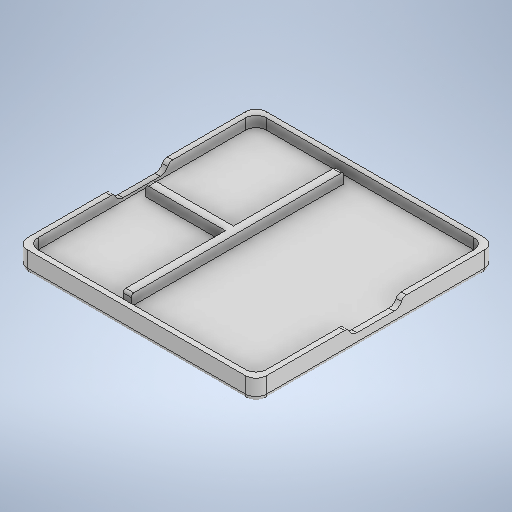
# Autodesk Inventor part: box-2
Saved by Autodesk Inventor 2025 (Build 290162000, 162)
## iProperties
Created: 2026-01-27
Part Number: box-2
Material: 一般
Document SubType Name: Modeling
Designer: mahhy
Density: 1 g/cm^3
Appearance: 既定
Author: mahhy
## iProperties of the stored document box-2_3D プリント.ipt
Created: 2026-01-27
Part Number: box-2_3D プリント
Material: 一般
Document SubType Name: Modeling
Designer: mahhy
Density: 1 g/cm^3
Appearance: 既定
Author: mahhy
Autodesk Inventor part; units mm, degrees
ref_plane "YZ Plane" through (0, 0, 0) normal (1, 0, 0) x (0, 1, 0)
ref_plane "XZ Plane" through (0, 0, 0) normal (0, 1, 0) x (-1, 0, 0)
ref_plane "XY Plane" through (0, 0, 0) normal (0, 0, 1) x (1, 0, 0)
sketch "底面スケッチ" plane through (0, 0, 0) normal (0, 1, 0) x (-1, 0, 0)
  line L0 (2, 0) -> (43, 0)
  line L1 (45, -2) -> (45, -43)
  line L2 (43, -45) -> (2, -45)
  line L3 (0, -43) -> (0, -2)
  arc A0 (45, -2) -> (43, 0) centre (43, -2) ccw
  arc A1 (43, -45) -> (45, -43) centre (43, -43) ccw
  arc A2 (0, -43) -> (2, -45) centre (2, -43) ccw
  arc A3 (2, 0) -> (0, -2) centre (2, -2) ccw
  point P0 (0, 0)
  point P1 (45, -45)
  point P2 (45, 0)
  point P3 (0, -45)
  dimension "d0" = 45
  dimension "d1" = 45
  dimension "d4" = 2
  constraints: 8 end point, 8 point on circle, 8 point on line, 8 tangent, 4 centre point, 3 equal radius, 2 parallel, 1 horizontal, 1 perpendicular
  measures "d0" distance of point (45, -45) point (0, -45)
  measures "d1" distance between parallel lines of L2 L0
  measures "d4" radius of A0
extrude "押し出し1" add sketch "底面スケッチ" along normal blind 4
sketch "スケッチ2" plane through (0, 4, 0) normal (0, 1, 0) x (1, 0, 0)
  line L0 (-42, 1) -> (-3, 1)
  line L1 (-1, 3) -> (-1, 42)
  line L2 (-3, 44) -> (-42, 44)
  line L3 (-44, 42) -> (-44, 3)
  line L4 (-2, 45) -> (-43, 45) projected
  line L5 (-43, 0) -> (-2, 0) projected
  line L6 (-45, 43) -> (-45, 2) projected
  line L7 (0, 2) -> (0, 43) projected
  arc A0 (-44, 3) -> (-42, 1) centre (-42, 3) ccw
  arc A1 (-3, 1) -> (-1, 3) centre (-3, 3) ccw
  arc A2 (-42, 44) -> (-44, 42) centre (-42, 42) ccw
  arc A3 (-1, 42) -> (-3, 44) centre (-3, 42) ccw
  point P0 (0, 0)
  dimension "d5" = 1
  dimension "d6" = 1
  dimension "d7" = 1
  dimension "d8" = 1
  dimension "d9" = 2
  constraints: 8 end point, 8 point on circle, 8 tangent, 4 centre point, 3 equal radius, 2 parallel, 1 horizontal, 1 perpendicular
  measures "d5" distance between parallel lines of L4 L2
  measures "d6" distance between parallel lines of L5 L0
  measures "d7" distance between parallel lines of L6 L3
  measures "d8" distance between parallel lines of L7 L1
  measures "d9" radius of A0
extrude "押し出し2" cut sketch "スケッチ2" against normal blind 2
sketch "スケッチ3" plane through (0, 2, 0) normal (0, 1, 0) x (1, 0, 0)
  line L0 (-3, 1) -> (-42, 1) projected
  line L1 (-42, 44) -> (-3, 44) projected
  line L2 (-44, 3) -> (-44, 42) projected
  line L3 (-27.5, 2.5) -> (-26, 2.5)
  line L4 (-26, 2.5) -> (-26, 42.5)
  line L5 (-26, 42.5) -> (-27.5, 42.5)
  line L6 (-27.5, 42.5) -> (-27.5, 2.5)
  line L7 (-1, 42) -> (-1, 3) projected
  line L8 (-27.5, 21.75) -> (-42.5, 21.75)
  line L9 (-42.5, 21.75) -> (-42.5, 23.25)
  line L10 (-42.5, 23.25) -> (-27.5, 23.25)
  line L11 (-27.5, 23.25) -> (-27.5, 21.75)
  point P0 (0, 0)
  point P1 (-26, 22.5)
  point P2 (-1, 22.5)
  point P3 (-42.5, 22.5)
  point P4 (-1, 22.5)
  dimension "d19" = 1.5
  dimension "d20" = 40
  dimension "d21" = 16.5
  dimension "d22" = 1.5
  dimension "d23" = 15
  constraints: 16 end point, 4 midpoint, 4 parallel, 2 horizontal, 2 horizontal alignment, 2 perpendicular, 1 point on line
  measures "d19" distance of L5.end L4.end
  measures "d20" distance of L3.end L4.end
  measures "d21" distance between parallel lines of L2 L6
  measures "d22" distance of L8.end L9.end
  measures "d23" distance of L9.end L10.end
extrude "押し出し3" add sketch "スケッチ3" along normal blind 2
fillet "フィレット1" radius 0.5 3 edges at (-26.75, 4, -42.5) (-26.75, 4, -2.5) (-42.5, 4, -22.5)
fillet "フィレット2" radius 1 8 edges at (-44.4142, 0, -44.4142) (-45, 0, -22.5) (-44.4142, 0, -0.5858) (-22.5, 0, 0) (-0.5858, 0, -0.5858) (0, 0, -22.5) (-0.5858, 0, -44.4142) (-22.5, 0, -45)
sketch "スケッチ4" plane through (0, 4, 0) normal (0, 1, 0) x (1, 0, 0)
  line L0 (-1, 42) -> (-1, 3) projected
  line L1 (-1, 27.5) -> (0, 27.5)
  line L2 (0, 27.5) -> (0, 17.5)
  line L3 (0, 17.5) -> (-1, 17.5)
  line L4 (-1, 17.5) -> (-1, 27.5)
  line L5 (0, 2) -> (0, 43) projected
  line L6 (-45, 2) -> (-45, 43) projected
  line L7 (-44, 43) -> (-44, 2) projected
  line L8 (-45, 27.5) -> (-44, 27.5)
  line L9 (-44, 27.5) -> (-44, 17.5)
  line L10 (-44, 17.5) -> (-45, 17.5)
  line L11 (-45, 17.5) -> (-45, 27.5)
  point P0 (0, 0)
  point P1 (0, 22.5)
  point P2 (0, 22.5)
  point P3 (-45, 22.5)
  point P4 (-44, 22.5)
  dimension "d24" = 10
  dimension "d25" = 10
  constraints: 16 end point, 4 midpoint, 4 parallel, 4 point on line, 2 horizontal, 2 perpendicular, 1 coincident, 1 horizontal alignment
  measures "d24" distance of L2.end L1.end
  measures "d25" distance between parallel lines of L10 L8
extrude "押し出し4" cut sketch "スケッチ4" against normal blind 1.5
fillet "フィレット3" radius 1.5 4 edges at (-44.5, 2.5, -27.5) (-44.5, 2.5, -17.5) (-0.5, 2.5, -27.5) (-0.5, 2.5, -17.5)
fillet "フィレット4" radius 1 8 edges at (-0.5, 3.9995, -27.5) (-0.5, 4, -27.5) (-0.5, 3.9995, -17.5) (-0.5, 4, -17.5) (-44.5, 4, -27.5) (-44.5, 3.9995, -27.5) (-44.5, 4, -17.5) (-44.5, 3.9995, -17.5)
equation "\"d1\" = d0"
equation "\"d6\" = d5"
equation "\"d7\" = d5"
equation "\"d8\" = d5"
equation "\"d25\" = d24"
